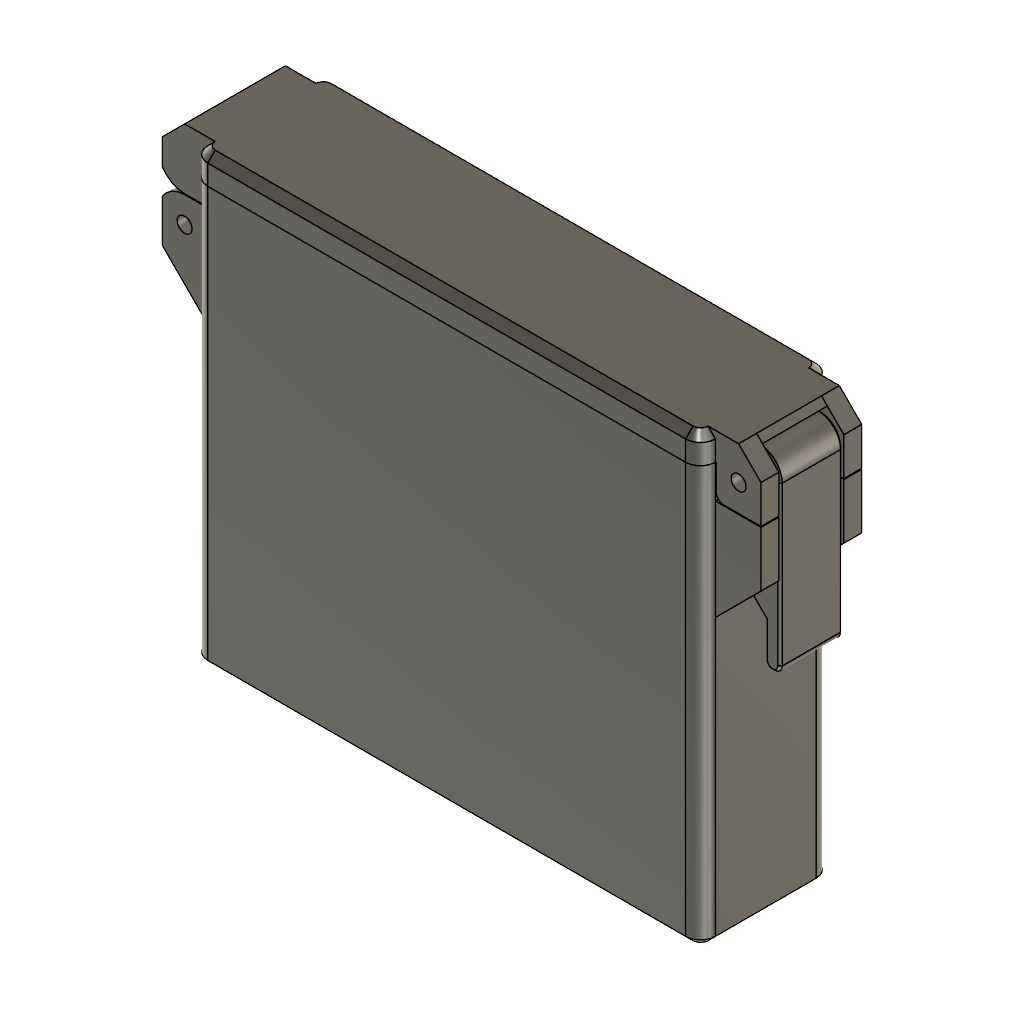
cartridge-template (Autodesk Fusion 360 design; units mm, degrees)
part number: 2026-09-30-10-10-59-994
part number: 2026-09-30-10-11-00-351
part number: 2026-09-30-10-20-21-039
part number: 2026-09-30-10-31-52-595
Autodesk Fusion 360 part; units mm, degrees
ref_plane "WorkPlane1" through (0, 0, 0) normal (0, 0, 1) x (1, 0, 0) in component "Body"
sketch "Body outline" plane through (0, 0, 0) normal (0, 0, 1) x (1, 0, 0) in component "Body"
  line L0 (-34, -8.75) -> (34, -8.75)
  line L1 (34, -8.75) -> (34, 8.75)
  line L2 (34, 8.75) -> (-34, 8.75)
  line L3 (-34, 8.75) -> (-34, -8.75)
  dimension "d14" = 34
  dimension "d15" = 8.75
  dimension "d16" = 34
  dimension "d17" = 8.75
  constraint horizontal L0
  constraint vertical L1
  constraint horizontal L2
  constraint vertical L3
  measures "d14" horizontal distance of origin L0.start
  measures "d15" vertical distance of origin L0.start
  measures "d16" horizontal distance of origin L1.end
  measures "d17" vertical distance of origin L1.end
extrude "Extrude1" add sketch "Body outline" along normal blind 56 makes body 1 in component "Body"
fillet "Fillet1" radius 2 4 edges at (-34, 8.75, 28) (34, 8.75, 28) (34, -8.75, 28) (-34, -8.75, 28) on bodies 1 in component "Body"
sketch "Tongue" plane through (0, 0, 56) normal (0, 0, 1) x (1, 0, 0) in component "Body"
  arc A0 (-34, -6.75) -> (-32, -8.75) centre (-32, -6.75) ccw
  line L0 (-32, -8.75) -> (32, -8.75)
  arc A1 (32, -8.75) -> (34, -6.75) centre (32, -6.75) ccw
  line L1 (34, -6.75) -> (34, 6.75)
  arc A2 (34, 6.75) -> (32, 8.75) centre (32, 6.75) ccw
  line L2 (32, 8.75) -> (-32, 8.75)
  arc A3 (-32, 8.75) -> (-34, 6.75) centre (-32, 6.75) ccw
  line L3 (-34, 6.75) -> (-34, -6.75)
  arc A4 (-32.8, -6.75) -> (-32, -7.55) centre (-32, -6.75) ccw
  line L4 (-32, -7.55) -> (32, -7.55)
  arc A5 (32, -7.55) -> (32.8, -6.75) centre (32, -6.75) ccw
  line L5 (32.8, -6.75) -> (32.8, 6.75)
  arc A6 (32.8, 6.75) -> (32, 7.55) centre (32, 6.75) ccw
  line L6 (32, 7.55) -> (-32, 7.55)
  arc A7 (-32, 7.55) -> (-32.8, 6.75) centre (-32, 6.75) ccw
  line L7 (-32.8, 6.75) -> (-32.8, -6.75)
  dimension "d22" = 1.2
extrude "Extrude2" add sketch "Tongue" along normal blind 1.5 contours A4 L4 A5 L5 A6 L6 A7 L7 bodies 1 in component "Body"
sketch "Hinge ear" plane through (0, 0, 0) normal (0, 1, 0) x (1, 0, 0) in component "Body"
  line L0 (-34, -51.5) -> (-37.1, -51.5)
  arc A0 (-40.1, -49.8028) -> (-37.1, -51.5) centre (-37.1, -48) ccw
  line L1 (-40.1, -49.8028) -> (-40.1, -44.1)
  line L2 (-40.1, -44.1) -> (-34, -38)
  line L3 (-34, -38) -> (-34, -51.5)
  circle A1 centre (-37.1, -48) radius 1
  dimension "d25" = 34
  dimension "d26" = 51.5
  dimension "d27" = 3.5
  dimension "d28" = 3.1
  dimension "d29" = 6.1
  dimension "d30" = 7.4
  dimension "d31" = 13.5
  dimension "d32" = 2
  constraint horizontal L0
  constraint tangent L0 A0
  constraint vertical L1
  constraint vertical L3
  constraint coincident A0.centre A1.centre
  measures "d25" horizontal distance of origin L0.start
  measures "d26" vertical distance of origin L0.start
  measures "d27" radius of A0
  measures "d28" horizontal distance of L0.start L0.end
  measures "d29" horizontal distance of L0.start A0.start
  measures "d30" vertical distance of L0.start L1.end
  measures "d31" vertical distance of L0.start L2.end
  measures "d32" diameter of A1
sketch "Latch post" plane through (0, 0, 0) normal (0, 1, 0) x (1, 0, 0) in component "Body"
  line L0 (34, -51.5) -> (40.1, -51.5)
  line L1 (40.1, -51.5) -> (40.1, -44.1)
  line L2 (40.1, -44.1) -> (34, -38)
  line L3 (34, -38) -> (34, -51.5)
  dimension "d33" = 34
  dimension "d34" = 51.5
  dimension "d35" = 6.1
  dimension "d36" = 7.4
  dimension "d37" = 13.5
  constraint horizontal L0
  constraint vertical L1
  constraint vertical L3
  measures "d33" horizontal distance of origin L0.start
  measures "d34" vertical distance of origin L0.start
  measures "d35" horizontal distance of L0.start L0.end
  measures "d36" vertical distance of L0.start L1.end
  measures "d37" vertical distance of L0.start L2.end
extrude "Extrude3" add sketch "Hinge ear" along normal blind 2.4 from surface at 4.35 bodies 1 in component "Body"
extrude "Extrude4" add sketch "Latch post" along normal blind 2.4 from surface at 4.35 bodies 1 in component "Body"
mirror "Mirror1" about plane through (0, 0, 0) normal (0, 1, 0) of "Extrude3", "Extrude4" in component "Body"
sketch "Catch bar" plane through (0, 0, 0) normal (0, 1, 0) x (1, 0, 0) in component "Body"
  line L0 (34, -49.2) -> (36.6, -49.2)
  arc A0 (36.6, -49.2) -> (37.6, -48.2) centre (36.6, -48.2) ccw
  line L1 (37.6, -48.2) -> (37.6, -44.1)
  arc A1 (37.6, -44.1) -> (35.4, -44.1) centre (36.5, -44.1) ccw
  line L2 (35.4, -44.1) -> (34, -44.1)
  line L3 (34, -44.1) -> (34, -49.2)
  dimension "d46" = 34
  dimension "d47" = 49.2
  dimension "d48" = 1
  dimension "d49" = 1.1
  dimension "d50" = 3.6
  dimension "d51" = 5.1
  constraint horizontal L0
  constraint vertical L1
  constraint tangent L0 A0
  constraint tangent A0 L1
  constraint tangent L1 A1
  constraint horizontal A1.end A1.centre
  constraint horizontal L2
  constraint vertical L3
  measures "d46" horizontal distance of origin L0.start
  measures "d47" vertical distance of origin L0.start
  measures "d48" radius of A0
  measures "d49" radius of A1
  measures "d50" horizontal distance of L0.start L1.end
  measures "d51" vertical distance of L0.start L2.end
extrude "Extrude5" add sketch "Catch bar" along normal mid plane 8.7 bodies 1 in component "Body"
ref_plane "WorkPlane1" through (0, 0, 57.7) normal (0, 0, 1) x (1, 0, 0) in component "Lid"
sketch "Lid outline" plane through (0, 0, 57.7) normal (0, 0, 1) x (1, 0, 0) in component "Lid"
  line L0 (-34, -8.75) -> (34, -8.75)
  line L1 (34, -8.75) -> (34, 8.75)
  line L2 (34, 8.75) -> (-34, 8.75)
  line L3 (-34, 8.75) -> (-34, -8.75)
  dimension "d56" = 34
  dimension "d57" = 8.75
  dimension "d58" = 34
  dimension "d59" = 8.75
  constraint horizontal L0
  constraint vertical L1
  constraint horizontal L2
  constraint vertical L3
  measures "d56" horizontal distance of origin L0.start
  measures "d57" vertical distance of origin L0.start
  measures "d58" horizontal distance of origin L1.end
  measures "d59" vertical distance of origin L1.end
extrude "Extrude1'" add sketch "Lid outline" along normal blind 2 separate body makes body 2 in component "Lid"
fillet "Fillet1'" radius 2 4 edges at (-34, 8.75, 58.7) (34, 8.75, 58.7) (34, -8.75, 58.7) (-34, -8.75, 58.7) on bodies 2 in component "Lid"
chamfer "Chamfer1" distance 1 angle 45 8 edges at (-33.4142, -8.1642, 59.7) (-34, 0, 59.7) (-33.4142, 8.1642, 59.7) (0, 8.75, 59.7) (33.4142, 8.1642, 59.7) (34, 0, 59.7) (33.4142, -8.1642, 59.7) (0, -8.75, 59.7) on bodies 2 in component "Lid"
sketch "Skirt" plane through (0, 0, 57.7) normal (0, 0, -1) x (-1, 0, 0) in component "Lid"
  arc A0 (32, -8.75) -> (34, -6.75) centre (32, -6.75) ccw
  line L0 (34, 6.75) -> (34, -6.75)
  arc A1 (34, 6.75) -> (32, 8.75) centre (32, 6.75) ccw
  line L1 (-32, 8.75) -> (32, 8.75)
  arc A2 (-32, 8.75) -> (-34, 6.75) centre (-32, 6.75) ccw
  line L2 (-34, -6.75) -> (-34, 6.75)
  arc A3 (-34, -6.75) -> (-32, -8.75) centre (-32, -6.75) ccw
  line L3 (32, -8.75) -> (-32, -8.75)
  arc A4 (32, -7.65) -> (32.9, -6.75) centre (32, -6.75) ccw
  line L4 (32.9, 6.75) -> (32.9, -6.75)
  arc A5 (32.9, 6.75) -> (32, 7.65) centre (32, 6.75) ccw
  line L5 (-32, 7.65) -> (32, 7.65)
  arc A6 (-32, 7.65) -> (-32.9, 6.75) centre (-32, 6.75) ccw
  line L6 (-32.9, -6.75) -> (-32.9, 6.75)
  arc A7 (-32.9, -6.75) -> (-32, -7.65) centre (-32, -6.75) ccw
  line L7 (32, -7.65) -> (-32, -7.65)
  dimension "d65" = 1.1
extrude "Extrude2'" add sketch "Skirt" along normal blind 1.7 bodies 2 in component "Lid"
sketch "Lid hinge cheeks" plane through (0, 0, 0) normal (0, 1, 0) x (1, 0, 0) in component "Lid"
  line L0 (-33, -59.7) -> (-37.1, -59.7)
  line L1 (-37.1, -59.7) -> (-40.1, -56.7)
  line L2 (-40.1, -56.7) -> (-40.1, -53.21)
  line L3 (-37.1, -51.6) -> (-34.1, -51.6)
  arc A0 (-37.1, -51.6) -> (-40.1, -53.21) centre (-37.1, -55.2) ccw
  line L4 (-34.1, -51.6) -> (-34.1, -56)
  line L5 (-34.1, -56) -> (-33, -56)
  line L6 (-33, -56) -> (-33, -59.7)
  dimension "d68" = 33
  dimension "d69" = 59.7
  dimension "d70" = 3.6
  dimension "d71" = 4.1
  dimension "d72" = 7.1
  dimension "d73" = 3
  dimension "d74" = 8.1
  dimension "d75" = 1.1
  dimension "d76" = 3.7
  constraint horizontal L0
  constraint vertical L2
  constraint horizontal L3
  constraint tangent L3 A0
  constraint vertical L4
  constraint horizontal L5
  constraint vertical L6
  constraint vertical L0.end L3.start
  measures "d68" horizontal distance of origin L0.start
  measures "d69" vertical distance of origin L0.start
  measures "d70" radius of A0
  measures "d71" horizontal distance of L0.start L0.end
  measures "d72" horizontal distance of L0.start L1.end
  measures "d73" vertical distance of L0.start L1.end
  measures "d74" vertical distance of L0.start L3.end
  measures "d75" horizontal distance of L0.start L3.end
  measures "d76" vertical distance of L0.start L4.end
extrude "Extrude3'" add sketch "Lid hinge cheeks" along normal mid plane 13.5 bodies 2 in component "Lid"
sketch "Lid hinge knuckle" plane through (0, 0, 0) normal (0, 1, 0) x (1, 0, 0) in component "Lid"
  line L0 (-33, -59.7) -> (-37.1, -59.7)
  line L1 (-37.1, -59.7) -> (-40.1, -56.7)
  line L2 (-40.1, -56.7) -> (-40.1, -48)
  arc A0 (-34.1, -48) -> (-40.1, -48) centre (-37.1, -48) ccw
  line L3 (-34.1, -48) -> (-34.1, -56)
  line L4 (-34.1, -56) -> (-33, -56)
  line L5 (-33, -56) -> (-33, -59.7)
  circle A1 centre (-37.1, -48) radius 1
  dimension "d79" = 33
  dimension "d80" = 59.7
  dimension "d81" = 4.1
  dimension "d82" = 7.1
  dimension "d83" = 3
  dimension "d84" = 1.1
  dimension "d85" = 3.7
  dimension "d86" = 11.7
  dimension "d87" = 2
  constraint horizontal L0
  constraint vertical L2
  constraint vertical L3
  constraint tangent L2 A0
  constraint tangent A0 L3
  constraint horizontal L4
  constraint vertical L5
  constraint coincident A0.centre A1.centre
  measures "d79" horizontal distance of origin L0.start
  measures "d80" vertical distance of origin L0.start
  measures "d81" horizontal distance of L0.start L0.end
  measures "d82" horizontal distance of L0.start L1.end
  measures "d83" vertical distance of L0.start L1.end
  measures "d84" horizontal distance of L0.start A0.start
  measures "d85" vertical distance of L0.start L3.end
  measures "d86" vertical distance of L0.start L2.end
  measures "d87" diameter of A1
extrude "Extrude4'" add sketch "Lid hinge knuckle" along normal mid plane 8.6 bodies 2 in component "Lid"
sketch "Lid latch lug" plane through (0, 0, 0) normal (0, 1, 0) x (1, 0, 0) in component "Lid"
  line L0 (33, -59.7) -> (37.1, -59.7)
  line L1 (37.1, -59.7) -> (40.1, -56.7)
  line L2 (40.1, -56.7) -> (40.1, -51.6)
  line L3 (40.1, -51.6) -> (35.1, -51.6)
  arc A0 (35.1, -51.6) -> (34.1, -52.6) centre (35.1, -52.6) ccw
  line L4 (34.1, -52.6) -> (34.1, -56)
  line L5 (34.1, -56) -> (33, -56)
  line L6 (33, -56) -> (33, -59.7)
  circle A1 centre (37.1, -55.2) radius 1
  point P0 (37.1, -55.2)
  dimension "d90" = 33
  dimension "d91" = 59.7
  dimension "d92" = 1
  dimension "d93" = 4.1
  dimension "d94" = 7.1
  dimension "d95" = 3
  dimension "d96" = 8.1
  dimension "d97" = 1.1
  dimension "d98" = 3.7
  dimension "d99" = 4.5
  dimension "d100" = 2
  constraint horizontal L0
  constraint vertical L2
  constraint horizontal L3
  constraint vertical L4
  constraint tangent L3 A0
  constraint tangent A0 L4
  constraint horizontal L5
  constraint vertical L6
  constraint vertical L0.end P0
  constraint coincident P0 A1.centre
  measures "d90" horizontal distance of origin L0.start
  measures "d91" vertical distance of origin L0.start
  measures "d92" radius of A0
  measures "d93" horizontal distance of L0.start L0.end
  measures "d94" horizontal distance of L0.start L1.end
  measures "d95" vertical distance of L0.start L1.end
  measures "d96" vertical distance of L0.start L2.end
  measures "d97" horizontal distance of L0.start A0.end
  measures "d98" vertical distance of L0.start L4.end
  measures "d99" vertical distance of L0.start P0
  measures "d100" diameter of A1
extrude "Extrude5'" add sketch "Lid latch lug" along normal blind 2.4 from surface at 4.35 bodies 2 in component "Lid"
mirror "Mirror1'" about plane through (0, 0, 0) normal (0, 1, 0) of "Extrude5'" in component "Lid"
sketch "Lid latch lip" plane through (0, 0, 0) normal (0, 1, 0) x (1, 0, 0) in component "Lid"
  line L0 (33, -59.7) -> (37.1, -59.7)
  line L1 (37.1, -59.7) -> (37.9, -58.9148)
  arc A0 (34, -57.3977) -> (37.9, -58.9148) centre (37.1, -55.2) ccw
  line L2 (34, -57.3977) -> (34, -56)
  line L3 (34, -56) -> (33, -56)
  line L4 (33, -56) -> (33, -59.7)
  dimension "d106" = 33
  dimension "d107" = 59.7
  dimension "d108" = 3.8
  dimension "d109" = 4.5
  dimension "d110" = 4.1
  dimension "d111" = 4.9
  dimension "d112" = 1
  dimension "d113" = 3.7
  constraint horizontal L0
  constraint vertical L2
  constraint horizontal L3
  constraint vertical L4
  constraint vertical L0.end A0.centre
  measures "d106" horizontal distance of origin L0.start
  measures "d107" vertical distance of origin L0.start
  measures "d108" radius of A0
  measures "d109" vertical distance of L0.start A0.centre
  measures "d110" horizontal distance of L0.start L0.end
  measures "d111" horizontal distance of L0.start L1.end
  measures "d112" horizontal distance of L0.start A0.start
  measures "d113" vertical distance of L0.start L2.end
extrude "Extrude6" add sketch "Lid latch lip" along normal mid plane 8.7 bodies 2 in component "Lid"
sketch "Buckle profile" plane through (0, 0, 0) normal (0, 1, 0) x (1, 0, 0) in component "Buckle"
  arc A0 (38.1, -52.3716) -> (40.1, -55.2) centre (37.1, -55.2) ccw
  line L0 (40.1, -39.02) -> (40.1, -55.2)
  line L1 (38.1, -52.3716) -> (38.1, -43.85)
  arc A1 (38.1, -43.85) -> (37.1, -42.85) centre (37.1, -43.85) ccw
  line L2 (37.1, -42.85) -> (36.08, -42.85)
  arc A2 (36.08, -42.85) -> (35.6277, -43.0558) centre (36.08, -43.45) ccw
  arc A3 (34.605, -42.1009) -> (35.6277, -43.0558) centre (35.1, -42.5958) ccw
  line L3 (34.605, -42.1009) -> (38.3929, -38.3129)
  arc A4 (40.1, -39.02) -> (38.3929, -38.3129) centre (39.1, -39.02) ccw
  circle A5 centre (37.1, -55.2) radius 1.1
  dimension "d117" = 3
  dimension "d118" = 37.1
  dimension "d119" = 55.2
  dimension "d120" = 1
  dimension "d121" = 0.6
  dimension "d122" = 0.7
  dimension "d123" = 1
  dimension "d124" = 2
  dimension "d125" = 12.35
  dimension "d126" = 16.18
  dimension "d127" = 1.02
  dimension "d128" = 2
  dimension "d129" = 2.2
  constraint vertical L0
  constraint vertical L1
  constraint horizontal L2
  constraint tangent A0 L0
  constraint tangent L1 A1
  constraint tangent A1 L2
  constraint tangent L2 A2
  constraint tangent A2 A3
  constraint tangent A3 L3
  constraint tangent L3 A4
  constraint tangent L0 A4
  constraint coincident A0.centre A5.centre
  measures "d117" radius of A0
  measures "d118" horizontal distance of origin A0.centre
  measures "d119" vertical distance of origin A0.centre
  measures "d120" radius of A1
  measures "d121" radius of A2
  measures "d122" radius of A3
  measures "d123" radius of A4
  measures "d124" horizontal distance of A0.end A0.start
  measures "d125" vertical distance of A1.end A0.centre
  measures "d126" vertical distance of L0.start A0.centre
  measures "d127" horizontal distance of L2.end A0.centre
  measures "d128" horizontal distance of A0.centre A3.centre
  measures "d129" diameter of A5
extrude "Extrude1''" add sketch "Buckle profile" along normal mid plane 8.4 separate body makes body 3 in component "Buckle"
chamfer "Bottom chamfer" distance 1 angle 45 8 edges at (-33.4142, -8.1642, 0) (0, -8.75, 0) (33.4142, -8.1642, 0) (34, 0, 0) (33.4142, 8.1642, 0) (0, 8.75, 0) (-33.4142, 8.1642, 0) (-34, 0, 0) on bodies 1 in component "Body"
sketch "Cartridge - Dimensioned pull tab" plane through (0, 0, 0) normal (0, 1, 0) x (1, 0, 0) in component "Buckle"
  line L0 (38.1, -40) -> (40.1, -40)
  line L1 (40.1, -40) -> (40.1, -34)
  arc A0 (40.1, -34) -> (38.1, -34) centre (39.1, -34) ccw
  line L2 (38.1, -34) -> (38.1, -40)
  dimension "d147" = 2
  dimension "d148" = 40.1
  dimension "d149" = 40
  dimension "d150" = 6
  constraint horizontal L0
  constraint vertical L1
  constraint vertical L2
  constraint tangent L1 A0
  constraint tangent A0 L2
  measures "d147" horizontal distance of L0.start L0.end
  measures "d148" horizontal distance of origin L0.end
  measures "d149" vertical distance of origin L0.end
  measures "d150" vertical distance of L0.end L1.end
extrude "Cartridge - Pull tab" add sketch "Cartridge - Dimensioned pull tab" along normal mid plane 8.4 bodies 3 in component "Buckle"
chamfer "Cartridge - Buckle edge comfort" distance 0.3 angle 45 22 edges at (40.1, 4.2, 44.6) (39.1, 4.2, 33) (38.1, 4.2, 36.3029) (36.3525, 4.2, 40.3533) (34.6223, 4.2, 43.1075) (35.8315, 4.2, 42.9039) (36.59, 4.2, 42.85) (37.8071, 4.2, 43.1429) (38.1, 4.2, 48.1108) (34.6505, 4.2, 56.9321) (36.0744, 4.2, 54.8022) (40.1, -4.2, 44.6) (34.6505, -4.2, 56.9321) (38.1, -4.2, 48.1108) (37.8071, -4.2, 43.1429) (36.59, -4.2, 42.85) (35.8315, -4.2, 42.9039) (34.6223, -4.2, 43.1075) (36.3525, -4.2, 40.3533) (38.1, -4.2, 36.3029) (39.1, -4.2, 33) (36.0744, -4.2, 55.5978) on bodies 3 in component "Buckle"
component "Body" placed x (1, 0, 0) y (0, 1, 0) z (0, 0, 1) at (0, 0, 0)
component "Lid" placed x (1, 0, 0) y (0, 1, 0) z (0, 0, 1) at (0, 0, 0)
component "Buckle" placed x (1, 0, 0) y (0, 1, 0) z (0, 0, 1) at (0, 0, 0)
equation "Length = 68 mm" comment "Body length, end face to end face (ears extra)"
equation "Width = 17.5 mm" comment "Body width"
equation "d14 = Length / 2"
equation "d15 = Width / 2"
equation "d16 = Length / 2"
equation "d17 = Width / 2"
equation "d18 = BodyHeight"
equation "d25 = Length / 2"
equation "d26 = BodyHeight - 4.5 mm"
equation "d32 = PinHole"
equation "d33 = Length / 2"
equation "d34 = BodyHeight - 4.5 mm"
equation "d38 = Width / 2 - 4.4 mm"
equation "d41 = Width / 2 - 4.4 mm"
equation "d46 = Length / 2"
equation "d47 = BodyHeight - 6.8 mm"
equation "d52 = Width - 8.8 mm"
equation "d54 = BodyHeight + 1.7 mm"
equation "d56 = Length / 2"
equation "d57 = Width / 2"
equation "d58 = Length / 2"
equation "d59 = Width / 2"
equation "d68 = Length / 2 - 1 mm"
equation "d69 = BodyHeight + 3.7 mm"
equation "d77 = Width - 4 mm"
equation "d79 = Length / 2 - 1 mm"
equation "d80 = BodyHeight + 3.7 mm"
equation "d87 = PinHole"
equation "d88 = Width - 8.9 mm"
equation "d90 = Length / 2 - 1 mm"
equation "d91 = BodyHeight + 3.7 mm"
equation "d100 = PinHole"
equation "d101 = Width / 2 - 4.4 mm"
equation "d106 = Length / 2 - 1 mm"
equation "d107 = BodyHeight + 3.7 mm"
equation "d114 = Width - 8.8 mm"
equation "PinHole = 2 mm" comment "Pin holes for 1.75 mm filament pins; buckle eye is PinHole + 0.2"
equation "d118 = Length / 2 + 3.1 mm"
equation "d119 = BodyHeight - 0.8 mm"
equation "d129 = PinHole + 0.2 mm"
equation "d130 = Width - 8.9 mm - BuckleExtra"
equation "HeightUnits = 8" comment "Cartridge template control"
equation "BodyHeight = HeightUnits * 7 mm" comment "Cartridge template control"
equation "BuckleExtra = 0.2 mm" comment "Cartridge template control"
equation "GripThickness = 2 mm" comment "Cartridge template control"
equation "d147 = GripThickness"
equation "d148 = Length / 2 + 6.1 mm"
equation "d149 = BodyHeight - 16 mm"
equation "d151 = Width - 8.9 mm - BuckleExtra"
named bodies: "Body", "Lid", "Buckle"
